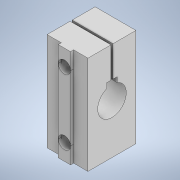
# Autodesk Inventor part: motor shaft clamp
Saved by Autodesk Inventor 2021 (Build 250183000, 183)
## iProperties
Created: 2022-09-09
Part Number: motor shaft clamp
Material: Generic
Document SubType Name: Modeling
Designer: szucs
Density: 1 g/cm^3
Appearance: Default
Author: szucs
Autodesk Inventor part; units mm, degrees
ref_plane "YZ Plane" through (0, 0, 0) normal (1, 0, 0) x (0, 1, 0)
ref_plane "XZ Plane" through (0, 0, 0) normal (0, 1, 0) x (-1, 0, 0)
ref_plane "XY Plane" through (0, 0, 0) normal (0, 0, 1) x (1, 0, 0)
sketch "Sketch1" plane through (0, 0, 0) normal (0, 0, 1) x (1, 0, 0)
  line L0 (0, 33.6) -> (0, -33.6) projected
  line L1 (-14, 0) -> (14, 0) projected
  line L2 (-10, 24) -> (10, 24)
  line L3 (10, 24) -> (10, -24)
  line L4 (10, -24) -> (-10, -24)
  line L5 (-10, -24) -> (-10, 24)
  point P0 (0, 0)
  dimension "d0" = 20
  dimension "d1" = 48
  constraints: 8 end point, 2 parallel, 1 horizontal, 1 perpendicular, 2 other
  measures "d0" distance of L3.end L4.end
  measures "d1" distance of L2.end L3.end
extrude "Extrusion1" add sketch "Sketch1" along normal blind 25
sketch "Sketch2" plane through (0, 0, 25) normal (0, 0, 1) x (1, 0, 0)
  line L0 (0, 49) -> (0, -49) projected
  line L1 (3, 35) -> (3, -35)
  line L2 (-3, 35) -> (-3, -35)
  line L3 (-10, -24) -> (10, -24) projected
  line L4 (10, -24) -> (10, 24) projected
  line L5 (10, 24) -> (-10, 24) projected
  line L6 (-10, 24) -> (-10, -24) projected
  point P0 (0, 0)
  point P1 (3, 24)
  point P2 (3, -24)
  point P3 (-3, -24)
  point P4 (-3, 24)
  dimension "d4" = 3
  dimension "d5" = 3
  constraints: 4 end point, 2 parallel
  measures "d4" distance between parallel lines of L0 L1
  measures "d5" distance between parallel lines of L0 L2
extrude "Extrusion2" cut sketch "Sketch2" against normal blind 1.5 contours L5 L4 L3 L1 | L2 L3 L6 L5
sketch "Sketch3" plane through (10, -24, 0) normal (1, 0, 0) x (0, 0, -1)
  line L0 (-23.5, 48) -> (-23.5, 0) projected
  line L1 (0, 0) -> (-23.5, 0) projected
  line L2 (0, 0) -> (0, 48) projected
  line L3 (0, 48) -> (-23.5, 48) projected
  line L4 (0, 0) -> (-23.5, 0) projected
  line L5 (-11.75, 0) -> (-11.75, 48)
  line L6 (0, 48) -> (-23.5, 48) projected
  line L7 (0, 24) -> (-23.5, 24)
  line L8 (-23.5, 0) -> (-23.5, 48) projected
  circle A0 centre (-11.75, 24) radius 7
  line L9 (-14.25, 28) -> (-9.25, 28)
  line L10 (-9.25, 28) -> (-9.25, 33)
  line L11 (-9.25, 33) -> (-14.25, 33)
  line L12 (-14.25, 33) -> (-14.25, 28)
  line L13 (-11.75, 17) -> (-11.75, 31)
  line L14 (-12.25, 0) -> (-12.25, 50)
  line L15 (-11.25, 0) -> (-11.25, 50)
  point P0 (-9.25, 30.5383)
  point P1 (-11.25, 33)
  point P2 (-11.25, 48)
  point P3 (-12.25, 48)
  point P4 (-12.25, 33)
  point P5 (-14.25, 30.5383)
  dimension "d8" = 14
  dimension "d9" = 5
  dimension "d10" = 5
  dimension "d11" = 11
  dimension "d12" = 0.5
  dimension "d13" = 0.5
  constraints: 18 end point, 4 midpoint, 4 parallel, 2 point on circle, 2 point on line, 1 centre point, 1 horizontal, 1 perpendicular, 1 other
  measures "d8" diameter of A0
  measures "d9" distance of L11.end L10.end
  measures "d10" distance of L10.end L9.end
  measures "d11" distance from line of L13.start L9
  measures "d12" distance between parallel lines of L5 L14
  measures "d13" distance between parallel lines of L5 L15
extrude "Extrusion3" cut sketch "Sketch3" against normal through all contours L3 L5 L11 L14 | A0 L12 L9 L14 L7 | L7 L14 A0 | L3 L15 L11 L5 | L14 A0 L12 L11 | L11 L5 A0 L14 | L14 L9 L5 L7 | L7 L5 A0 L14 | A0 L14 L9 L12 | L11 L15 A0 L5 | A0 L5 L9 L14 | L7 L15 A0 L5 | L5 L9 L15 L7 | L11 L10 A0 L15 | A0 L15 L9 L5 | L15 L9 L10 A0 L7 | L7 A0 L15 | A0 L10 L9 L15
sketch "Sketch4" plane through (0, 0, 25) normal (0, 0, 1) x (1, 0, 0)
  line L0 (3, -24) -> (3, 24) projected
  line L1 (3, 24) -> (-3, 24) projected
  line L2 (-3, 24) -> (-3, -24) projected
  line L3 (-3, -24) -> (3, -24) projected
  line L4 (0, 35) -> (0, -35) projected
  circle A0 centre (0, 16) radius 3
  circle A1 centre (0, -16) radius 3
  line L5 (-10, 6.5383) -> (-10, 9) projected
  line L6 (10, 6.5383) -> (-10, 6.5383) projected
  line L7 (10, 9) -> (10, 6.5383) projected
  line L8 (10, 9) -> (-10, 9) projected
  line L9 (10, 6.5383) -> (-10, 6.5383) projected
  line L10 (10, -7) -> (-10, -7) projected
  line L11 (-10, 6.5383) -> (-10, 6.5383) projected
  line L12 (10, 6.5383) -> (-10, 6.5383) projected
  line L13 (10, 6.5383) -> (10, 6.5383) projected
  line L14 (10, 6.5383) -> (-10, 6.5383) projected
  line L15 (10, 6.5383) -> (10, -7) projected
  line L16 (-10, -7) -> (-10, 6.5383) projected
  point P0 (0, 0)
  dimension "d16" = 6
  dimension "d17" = 6
  dimension "d18" = 8
  dimension "d19" = 8
  constraints: 2 centre point, 2 point on line
  measures "d16" diameter of A0
  measures "d17" diameter of A1
  measures "d18" distance from line of L1 A0.centre
  measures "d19" distance from line of L3 A1.centre
extrude "Extrusion4" cut sketch "Sketch4" against normal through all contours A1 L4 | L4 A1 | A0 L4 | L4 A0
body "Solid1"
